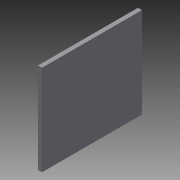
# Autodesk Inventor part: schreibtischplatte
Saved by Autodesk Inventor 2013 (Build 170138000, 138)
## iProperties
Created: 2014-03-29
Part Number: schreibtischplatte
Material: Generic
Document SubType Name: Modeling
Designer: hhanff
Density: 1 g/cm^3
Author: hhanff
Autodesk Inventor part; units mm, degrees
ref_plane "YZ Plane" through (0, 0, 0) normal (1, 0, 0) x (0, 1, 0)
ref_plane "XZ Plane" through (0, 0, 0) normal (0, 1, 0) x (-1, 0, 0)
ref_plane "XY Plane" through (0, 0, 0) normal (0, 0, 1) x (1, 0, 0)
sketch "Sketch1" plane through (0, 0, 0) normal (1, 0, 0) x (0, 1, 0)
  line L0 (0, 0) -> (552, 0)
  line L1 (552, 0) -> (552, 500)
  line L2 (552, 500) -> (0, 500)
  line L3 (0, 500) -> (0, 0)
  dimension "d0" = 552
  dimension "d2" = 500
  constraints: 8 end point, 2 parallel, 1 horizontal, 1 perpendicular
  measures "d0" distance of L1.end L2.end
  measures "d2" distance of L2.end L0.start
extrude "Extrusion1" add sketch "Sketch1" along normal blind 22
body "Solid1"
